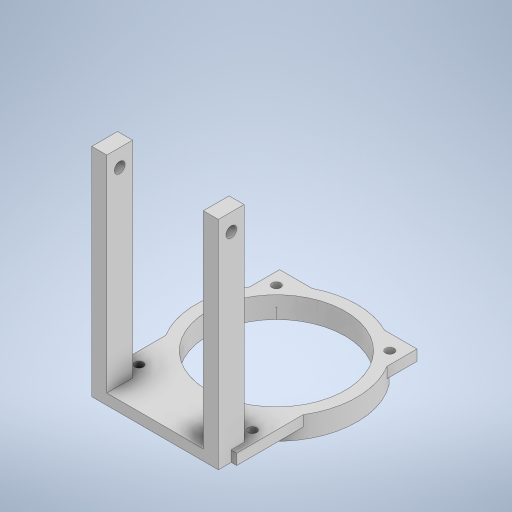
# Autodesk Inventor part: m500 thermal bracket
Saved by Autodesk Inventor 2023 (Build 270158000, 158)
## iProperties
Created: 2022-07-20
Part Number: m500 thermal bracket
Material: Generic
Document SubType Name: Modeling
Designer: Eli
Density: 1 g/cm^3
Appearance: Default
Author: Eli
Autodesk Inventor part; units mm, degrees
ref_plane "YZ Plane" through (0, 0, 0) normal (1, 0, 0) x (0, 1, 0)
ref_plane "XZ Plane" through (0, 0, 0) normal (0, 1, 0) x (-1, 0, 0)
ref_plane "XY Plane" through (0, 0, 0) normal (0, 0, 1) x (1, 0, 0)
sketch "Sketch1" plane through (0, 0, 0) normal (0, 1, 0) x (-1, 0, 0)
  line L0 (0, 0) -> (-40.64, 0)
  line L1 (-40.64, 0) -> (-40.64, -53.34)
  line L2 (-40.64, -53.34) -> (0, -53.34)
  line L3 (0, -53.34) -> (0, 0)
  circle A0 centre (-20.32, -32.0802) radius 20.32
  circle A1 centre (-20.32, -32.0802) radius 23.8125
  circle A2 centre (-3.556, -48.8442) radius 1.27
  circle A3 centre (-37.084, -48.8442) radius 1.27
  circle A4 centre (-37.084, -8.2042) radius 1.27
  circle A5 centre (-3.556, -8.2042) radius 1.27
  line L4 (-20.32, 0) -> (-20.32, -32.0802) construction
  point P0 (-40.64, -19.6652)
  point P1 (-40.64, -44.4952)
  point P2 (-31.0464, -53.34)
  point P3 (-9.5936, -53.34)
  point P4 (0, -44.4952)
  point P5 (0, -19.6652)
  dimension "d51" = 53.34
  dimension "d52" = 40.64
  dimension "d53" = 40.64
  dimension "d54" = 47.625
  dimension "d57" = 33.528
  dimension "d58" = 40.64
  dimension "d59" = 2.54
  dimension "d60" = 8.2042
  dimension "d63" = 32.0802
  constraints: 10 end point, 6 centre point, 3 equal radius, 2 coincident, 2 horizontal alignment, 2 parallel, 2 vertical alignment, 1 midpoint, 1 symmetric about line, 1 vertical
  measures "d51" distance of L0.end L1.end
  measures "d52" distance of L1.end L2.end
  measures "d53" diameter of A0
  measures "d54" diameter of A1
  measures "d57" distance of A3.centre A2.centre
  measures "d58" distance of A4.centre A3.centre
  measures "d59" diameter of A2
  measures "d60" distance from line of L0 A5.centre
  measures "d63" distance of L4.start L4.end
extrude "Extrusion1" add sketch "Sketch1" along normal blind 3.175 contours L3 A1 L1 L0 | A1 L3 | L3 A0 L1 A1 | L1 A1 | L3 A1 A2 L2 A3 L1 A0 | A1 A3 L2 L1 | L3 L2 A1 A2 | L2 A1
sketch "Sketch2" plane through (0, 3.175, 0) normal (0, 1, 0) x (1, 0, 0)
  line L0 (1.6002, 0) -> (39.0398, 0)
  line L1 (39.0398, 0) -> (39.0398, 3.81)
  line L2 (39.0398, 3.81) -> (1.6002, 3.81)
  line L3 (1.6002, 3.81) -> (1.6002, 0)
  line L4 (6.0452, 3.81) -> (6.0452, 0)
  line L5 (1.6002, 0) -> (39.0398, 0)
  line L6 (34.5948, 3.81) -> (34.5948, 0)
  line L7 (20.32, 3.81) -> (20.32, 0) construction
  circle A0 centre (20.32, 32.0802) radius 20.32 construction
  line L8 (20.32, 52.4002) -> (20.32, 32.0802) construction
  point P0 (34.5948, 0)
  point P1 (6.0452, 0)
  point P2 (20.32, 1.905)
  point P3 (6.0452, 1.905)
  dimension "d68" = 14.2748
  dimension "d69" = 4.445
  dimension "d70" = 3.81
  constraints: 18 end point, 4 midpoint, 4 point on line, 2 parallel, 1 collinear, 1 vertical, 1 vertical alignment, 2 other
  measures "d68" distance of point (20.32, 1.905) point (6.045, 1.905)
  measures "d69" distance between parallel lines of L4 L3
  measures "d70" distance between parallel lines of L2 L0
extrude "Extrusion2" add sketch "Sketch2" along normal blind 60.96 contours L3 L2 L4 L0 | L6 L2 L1 L0
sketch "Sketch10" plane through (0, 0, 0) normal (0, -1, 0) x (1, 0, 0)
  circle A0 centre (20.32, -32.0802) radius 20.32 construction
  line L0 (20.32, -52.4002) -> (20.32, -32.0802) construction
  circle A1 centre (20.32, -32.0802) radius 20.32
  circle A2 centre (37.084, -48.8442) radius 1.27 projected
  circle A3 centre (37.084, -48.8442) radius 3.3879
  circle A4 centre (3.556, -48.8442) radius 1.27 projected
  circle A5 centre (3.556, -48.8442) radius 3.3879
  circle A6 centre (20.32, -32.0802) radius 23.8125
  line L1 (33.6961, -12.3796) -> (6.9439, -12.3796)
  line L2 (6.9439, -12.3796) -> (6.9439, -3.5159)
  line L3 (6.9439, -3.5159) -> (33.6961, -3.5159)
  line L4 (33.6961, -3.5159) -> (33.6961, -12.3796)
  point P0 (0, 0)
  point P1 (34.6884, -46.4486)
  point P2 (39.3806, -46.3536)
  point P3 (6.9439, -12.3796)
  point P4 (1.2594, -46.3536)
  point P5 (5.9516, -46.4486)
  point P6 (6.0466, -51.1408)
  point P7 (34.5934, -51.1408)
  constraints: 10 end point, 4 coincident, 3 centre point, 2 parallel, 2 tangent, 1 horizontal, 1 perpendicular, 1 vertical, 1 vertical alignment, 5 other
extrude "Extrusion5" add sketch "Sketch10" along normal blind 3.175 contours A1 L1 A6 A3 | A1 L1 A6 | A3 A6 A5 A1 | A1 A5 A6 L1 | A6 L2 L3 L4
sketch "Sketch11" plane through (0, 0, 0) normal (0, 0, 1) x (1, 0, 0)
  line L0 (1.6002, 64.135) -> (6.0452, 64.135) projected
  line L1 (1.6002, 64.135) -> (39.0398, 64.135)
  line L2 (39.0398, 64.135) -> (39.0398, 0)
  line L3 (39.0398, 0) -> (1.6002, 0)
  line L4 (1.6002, 0) -> (1.6002, 64.135)
  line L5 (39.0398, 3.175) -> (39.0398, 64.135) construction
  line L6 (39.0398, 3.175) -> (39.0398, 0) construction
  line L7 (40.64, 0) -> (33.6961, 0) construction
  line L8 (34.5948, 3.175) -> (34.5948, 64.135) projected
  line L9 (6.0452, 64.135) -> (34.5948, 64.135)
  line L10 (34.5948, 64.135) -> (34.5948, 3.175)
  line L11 (34.5948, 3.175) -> (6.0452, 3.175)
  line L12 (6.0452, 3.175) -> (6.0452, 64.135)
  point P0 (0, 0)
  constraints: 18 end point, 4 parallel, 2 horizontal, 2 perpendicular, 1 point on line, 1 vertical
extrude "Extrusion6" add sketch "Sketch11" along normal blind 3.81 contours L0 L12 L11 L8 L1 L2 L3 L4
sketch "Sketch12" plane through (39.0398, 3.175, 0) normal (1, 0, 0) x (0, 0, -1)
  line L0 (3.81, 60.96) -> (-3.81, 60.96) construction
  line L1 (0, 60.96) -> (0, 55.88) construction
  point P0 (0, -3.175)
  dimension "d73" = 5.08
  constraints: 2 end point, 1 coincident, 1 midpoint, 1 vertical
  measures "d73" distance of L1.start L1.end
hole "Hole4" at (39.0398, 59.055, 0) direction (-1, 0, 0) diameter 3.175 depth 37.4396
body "Solid1"
